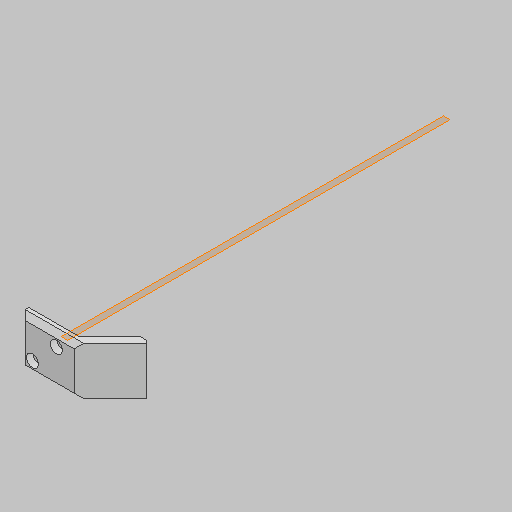
# Autodesk Inventor part: SoporteKlipperScreen
Saved by Autodesk Inventor 2025.4 (Build 294407000, 407)
## iProperties
Created: 2025-11-09
Part Number: SoporteKlipperScreen
Material: Genérico
Document SubType Name: Chapa
Designer: Inema
Density: 1 g/cm^3
Sheet Metal Rule: Por defecto_mm
Appearance: Valor por defecto
Author: Inema
Autodesk Inventor part; units mm, degrees
ref_plane "YZ Plane" through (0, 0, 0) normal (1, 0, 0) x (0, 1, 0)
ref_plane "XZ Plane" through (0, 0, 0) normal (0, 1, 0) x (-1, 0, 0)
ref_plane "XY Plane" through (0, 0, 0) normal (0, 0, 1) x (1, 0, 0)
ref_plane "Plano de trabajo1" through (19.2, 96.5, -0.8) normal (0, 1, 0) x (0, 0, -1)
sketch "Boceto1" plane through (19.2, 96.5, -0.8) normal (0, 1, 0) x (0, 0, -1)
  line L0 (-0.8, -18.4634) -> (-0.8, 18.4634) projected
  line L1 (-6.9748, 20) -> (-6.9748, -22)
  line L2 (-6.9748, -22) -> (21.3095, -50.2842)
  line L3 (-6.1748, 20) -> (283.8252, 20) projected
  line L4 (16.3598, -55.234) -> (-13.9748, -24.8995)
  line L5 (-13.9748, -24.8995) -> (-13.9748, 20)
  line L6 (21.3095, -50.2842) -> (16.3598, -55.234)
  line L7 (-6.9748, 20) -> (-13.9748, 20)
  point P0 (-0.8, 19.2)
  point P1 (-0.8, 18.4634)
  dimension "d0" = 135
  dimension "d1" = 42
  dimension "d2" = 40
  dimension "d3" = 7
  constraints: 12 end point, 1 horizontal, 1 horizontal alignment, 1 vertical, 1 other
  measures "d0" angle of L0 L2
  measures "d1" distance of L1.start L1.end
  measures "d2" distance of L1.end L2.end
  measures "d3" distance between parallel lines of L2 L4
extrude "Extrusión1" add sketch "Boceto1" against normal blind 40
chamfer "Chaflán1" distance 4 angle 45 1 edges at (69.4842, 76.5, -22.1095)
chamfer "Chaflán2" distance 4 angle 45 3 edges at (-0.8, 76.5, 13.1748) (21.6497, 96.5, 13.1748) (21.6497, 56.5, 13.1748)
sketch "Boceto2" plane through (3.2, 92.5, 13.1748) normal (0, 0, 1) x (1, 0, 0)
  circle A0 centre (6, -6) radius 2.5 projected
  circle A1 centre (26, -5.9999) radius 2.6 projected
  circle A2 centre (6, -26) radius 2.5 projected
  point P0 (-3.2, -92.5)
hole "Agujero1" at (29.2, 86.5001, 13.1748) at (9.2, 66.5, 13.1748) direction (0, 0, -1) diameter 5.5 end through all counterbore diameter 10 counterbore depth 5.5 clearance for "Tornillo de cabeza hueca DIN EN ISO 4762" size "M5" standard "DIN"
sketch "Boceto3" plane through (74.434, 56.5, -17.1598) normal (0.7071, 0, 0.7071) x (0.7071, 0, -0.7071)
  line L0 (114.1005, 77) -> (-42.8995, 77)
  line L1 (-42.8995, 77) -> (-42.8995, 0)
  line L2 (-42.8995, 0) -> (114.1005, 0)
  line L3 (114.1005, 0) -> (114.1005, 77)
  line L4 (-42.8995, 36) -> (-42.8995, 4) projected
  line L5 (0, 0) -> (-37.2426, 0) projected
  point P0 (-64.7666, -56.5)
  dimension "d19" = 157
  dimension "d20" = 77
  constraints: 8 end point, 2 collinear, 2 parallel, 1 horizontal, 1 perpendicular
  measures "d19" distance of L0.start L0.end
  measures "d20" distance of L0.end L1.end
extrude "Extrusión2" [suppressed]
equation "\"d17\" = Grosor"
equation "\"Profundidad_desahogo_plegado\" = 0.5 * Grosor"
equation "\"Grosor\" = 10"
